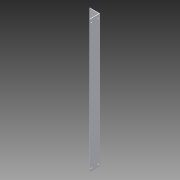
# Autodesk Inventor part: 26in Angle Channel CIM Mount Right
Saved by Autodesk Inventor 2013 (Build 170138000, 138)
## iProperties
Created: 2013-01-27
Part Number: 26in Angle Channel CIM Mount Right
Material: Aluminum 6061
Document SubType Name: Modeling
Designer: Naphat
Density: 1 g/cm^3
Author: Naphat
Autodesk Inventor part; units mm, degrees
ref_plane "YZ Plane" through (0, 0, 0) normal (1, 0, 0) x (0, 1, 0)
ref_plane "XZ Plane" through (0, 0, 0) normal (0, 1, 0) x (-1, 0, 0)
ref_plane "XY Plane" through (0, 0, 0) normal (0, 0, 1) x (1, 0, 0)
sketch "Sketch1" plane through (0, 0, 0) normal (0, 1, 0) x (-1, 0, 0)
  line L0 (0, 0) -> (50, 0)
  line L1 (50, 0) -> (50, 3)
  line L2 (0, 0) -> (0, 50)
  line L3 (0, 50) -> (3, 50)
  line L4 (3, 50) -> (3, 3)
  line L5 (3, 3) -> (50, 3)
  dimension "d0" = 50
  dimension "d1" = 3
  dimension "d2" = 50
  dimension "d3" = 3
  constraints: 12 end point, 3 perpendicular, 2 parallel, 1 horizontal
  measures "d0" distance of L0.start L0.end
  measures "d1" distance of L0.end L1.end
  measures "d2" distance of L0.start L2.end
  measures "d3" distance of L2.end L3.end
extrude "Extrusion1" add sketch "Sketch1" along normal blind 660.4
sketch "Sketch7" plane through (0, 0, 50) normal (1, 0, 0) x (0, 0, -1)
  line L0 (0, 0) -> (50, 0) projected
  line L1 (50, 0) -> (50, 660.4) projected
  line L2 (0, 660.4) -> (50, 660.4) projected
  line L3 (0, 0) -> (0, 660.4) projected
  circle A0 centre (6.35, 16) radius 3.175
  circle A1 centre (40.65, 16) radius 3.175
  circle A2 centre (6.35, 644.4) radius 3.175
  circle A3 centre (40.65, 644.4) radius 3.175
  line L4 (47, 0) -> (47, 660.4) construction
  dimension "d80" = 16
  dimension "d82" = 6.35
  dimension "d83" = 6.35
  dimension "d84" = 6.35
  dimension "d85" = 6.35
  dimension "d86" = 6.35
  dimension "d88" = 6.35
  dimension "d89" = 16
  dimension "d97" = 3
  dimension "d98" = 6.35
  constraints: 4 centre point, 2 end point, 2 horizontal alignment, 2 point on line, 2 vertical alignment, 1 perpendicular
  measures "d80" distance from line of L0 A0.centre
  measures "d82" distance from line of L3 A0.centre
  measures "d83" diameter of A0
  measures "d84" diameter of A1
  measures "d85" diameter of A2
  measures "d86" diameter of A3
  measures "d88" distance from line of L3 A2.centre
  measures "d89" distance from line of L2 A3.centre
  measures "d97" distance between parallel lines of L1 L4
  measures "d98" distance from line of A1.centre L4
hole "Hole1" at (0, 16, 43.65) at (0, 16, 9.35) at (0, 644.4, 43.65) at (0, 644.4, 9.35) direction (-1, 0, 0) diameter 6.35 depth 3 tip angle 118
equation "\"d84\" = d83"
equation "\"d85\" = d83"
equation "\"d86\" = d83"
body "Solid1"
